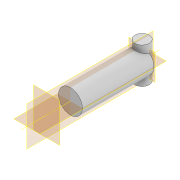
# Autodesk Inventor part: LowerarmY
Saved by Autodesk Inventor 2021 (Build 250183000, 183)
## iProperties
Created: 2020-12-19
Part Number: LowerarmY
Material: 一般
Document SubType Name: Modeling
Designer: Tazaki
Density: 3.02353 g/cm^3
Appearance: 既定
Mass: 1000 g
Surface Area: 316.951 cm^2
Volume: 330.739 cm^3
Author: Tazaki
Autodesk Inventor part; units mm, degrees
ref_plane "作業平面1" through (0, 0, -200) normal (0, 0, 1) x (1, 0, 0)
sketch "スケッチ3" plane through (0, 0, 0) normal (0, 0, 1) x (1, 0, 0)
  circle A0 centre (0, 0) radius 25
  dimension "d7" = 50
  constraints: 1 centre point, 1 coincident
  measures "d7" diameter of A0
extrude "押し出し2" add sketch "スケッチ3" against normal blind 200
sketch "スケッチ4" plane through (0, 0, 0) normal (0, 1, 0) x (-1, 0, 0)
  line L0 (71.1625, -50) -> (-59.4219, -50)
  line L1 (-59.4219, -50) -> (-59.4219, 51.3951)
  line L2 (-59.4219, 51.3951) -> (71.1625, 51.3951)
  line L3 (71.1625, 51.3951) -> (71.1625, -50)
  line L4 (-85.5387, 0) -> (97.2793, 0) projected
  point P0 (0, 0)
  dimension "d10" = 50
  constraints: 8 end point, 2 parallel, 1 horizontal, 1 perpendicular
  measures "d10" distance between parallel lines of L4 L0
extrude "押し出し3" cut sketch "スケッチ4" against normal mid plane 200
sketch "スケッチ5" plane through (0, 0, 0) normal (0, 1, 0) x (-1, 0, 0)
  circle A0 centre (0, -200) radius 15
  line L0 (-35, 0) -> (35, 0) projected
  point P0 (0, 0)
  dimension "d13" = 30
  dimension "d14" = 200
  constraints: 1 centre point, 1 vertical alignment
  measures "d13" diameter of A0
  measures "d14" distance from line of L0 A0.centre
extrude "押し出し4" add sketch "スケッチ5" along normal mid plane 75
